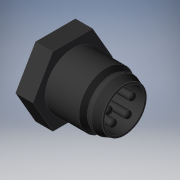
# Autodesk Inventor part: SCHUNK-SNT016581 Stecker EGP
Saved by Autodesk Inventor 2019 (Build 230136000, 136)
## iProperties
Created: 2022-08-29
Part Number: SCHUNK-SNT016581 Stecker EGP
Material: Generic
Catalog Web Link: www.cadenas.de
Description: EGP-Electrical 2-finger parallel gripper
Vendor: SCHUNK
Document SubType Name: Modeling
Designer: psAdmin
Manufacturer: SCHUNK
Mass: 0.444705 g
Surface Area: 5.81753 cm^2
Volume: 0.444705 cm^3
Density: 1 g/cm^3
Appearance: PSOLRGB-175-175-175
Category: PARTsolutions
Company: SCHUNK
Title: SCHUNK-SNT016581 Stecker EGP
Author: Cadenas PARTsolutions
Comments: Electrical 2-finger parallel gripper
PSOL_IDENT_0: {$CADENAS_DATA/23d-libs/schunk/greifsysteme/greifmodule/greifmodule_elektrisch/2_finger_parallelgrei
PSOL_IDENT_1: fer/kleinteilegreifer/egp/egp_stecker.prj},193 {VTYP=3D},{NB=SCHUNK-SNT016581 Stecker EGP},{LINA=SCH
PSOL_IDENT_2: UNK-SNT016581 Stecker EGP},{NN=EGP},{DATE=27.06.2022 11:10:53},{GEOMDATE=04.12.2019 08:06:16},{VERSI
PSOL_IDENT_3: ON=},{LINEID=10},{WBVAR=},{WBNUMERIC=}  {NB=SCHUNK-SNT016581 Stecker EGP},{LINA=SCHUNK-SNT016581 Ste
PSOL_IDENT_4: cker EGP},{KT=DUMMY},{IDNR=SNT016581},{TYP=EGP}
NB: SCHUNK-SNT016581 Stecker EGP
NN: EGP
NT: Electrical 2-finger parallel gripper
NBSYN: SCHUNK-$IDNR. Stecker $TYP.
LINA: SCHUNK-SNT016581 Stecker EGP
CATALOG: SCHUNK
IDNR: SNT016581
TYP: EGP
SUPPLIER: SCHUNK
ARTICLENO: SCHUNK-SNT016581 Stecker EGP
BOMINFO: SCHUNK-SNT016581 Stecker EGP
CREATOR: CADENAS GmbH
Autodesk Inventor part; units mm, degrees
sketch "Sketch_1" plane through (0, 0, 0) normal (0, 0, 1) x (1, 0, 0)
  line L0 (10, 0) -> (0, 0)
  line L1 (0, 0) -> (0, 6)
  line L2 (0, 6) -> (2.5, 6)
  line L3 (2.5, 6) -> (2.5, 4)
  line L4 (2.5, 4) -> (7.4, 4)
  line L5 (7.4, 4) -> (8, 3.4)
  line L6 (8, 3.4) -> (8.5, 3.4)
  line L7 (8.5, 3.4) -> (8.5, 3.6)
  line L8 (8.5, 3.6) -> (8.8, 3.6)
  line L9 (8.8, 3.6) -> (9.9, 3.2)
  line L10 (9.9, 3.2) -> (10, 3.2)
  line L11 (10, 3.2) -> (10, 2.9)
  line L12 (10, 2.9) -> (5, 2.9)
  line L13 (5, 2.9) -> (5, 0)
  line L14 (5, 0) -> (0, 0)
  constraints: 30 end point
revolve "Revolution1" add sketch "Sketch_1" angle 360 about axis through (10, 0, 0) along (1, 0, 0)
sketch "Sketch_2" plane through (0, 0, 0) normal (1, 0, 0) x (0, 1, 0)
  circle A0 centre (0, 0) radius 20
  line L0 (0, 5.7735) -> (-5, 2.8868)
  line L1 (-5, 2.8868) -> (-5, -2.8868)
  line L2 (-5, -2.8868) -> (0, -5.7735)
  line L3 (0, -5.7735) -> (5, -2.8868)
  line L4 (5, -2.8868) -> (5, 2.8868)
  line L5 (5, 2.8868) -> (0, 5.7735)
  constraints: 12 end point, 1 centre point
extrude "Extrusion1" cut sketch "Sketch_2" along normal blind 2.5
sketch "Sketch_3" plane through (0, 0, 1.7) normal (0, 0, 1) x (1, 0, 0)
  line L0 (9.8, 0.5) -> (5, 0.5)
  line L1 (5, 0.5) -> (5, 1)
  line L2 (5, 1) -> (9.3, 1)
  arc A0 (9.8, 0.5) -> (9.3, 1) centre (9.3, 0.5) ccw
  line L3 (9.8, 0.5) -> (5, 0.5)
  constraints: 8 end point, 2 point on circle, 1 centre point
revolve "Revolution2" add sketch "Sketch_3" angle 360 about axis through (9.8, 0.5, 1.7) along (1, 0, 0)
sketch "Pins_SKETCH_1" plane through (0, 0, -1.7) normal (0, 0, 1) x (1, 0, 0)
  line L0 (9.8, 0.5) -> (5, 0.5)
  line L1 (5, 0.5) -> (5, 1)
  line L2 (5, 1) -> (9.3, 1)
  arc A0 (9.8, 0.5) -> (9.3, 1) centre (9.3, 0.5) ccw
  line L3 (9.8, 0.5) -> (5, 0.5)
  constraints: 8 end point, 2 point on circle, 1 centre point
sketch "Pins_SKETCH_2" plane through (0, -1.95, -1.075) normal (0, 0, 1) x (1, 0, 0)
  line L0 (9.8, 0.5) -> (5, 0.5)
  line L1 (5, 0.5) -> (5, 1)
  line L2 (5, 1) -> (9.3, 1)
  arc A0 (9.8, 0.5) -> (9.3, 1) centre (9.3, 0.5) ccw
  line L3 (9.8, 0.5) -> (5, 0.5)
  constraints: 8 end point, 2 point on circle, 1 centre point
sketch "Pins_SKETCH_3" plane through (0, -1.95, 1.075) normal (0, 0, 1) x (1, 0, 0)
  line L0 (9.8, 0.5) -> (5, 0.5)
  line L1 (5, 0.5) -> (5, 1)
  line L2 (5, 1) -> (9.3, 1)
  arc A0 (9.8, 0.5) -> (9.3, 1) centre (9.3, 0.5) ccw
  line L3 (9.8, 0.5) -> (5, 0.5)
  constraints: 8 end point, 2 point on circle, 1 centre point
revolve "Revolution3" add sketch "Pins_SKETCH_1" angle 360 about axis through (9.8, 0.5, -1.7) along (1, 0, 0)
revolve "Revolution4" add sketch "Pins_SKETCH_2" angle 360 about axis through (9.8, -1.45, -1.075) along (1, 0, 0)
revolve "Revolution5" add sketch "Pins_SKETCH_3" angle 360 about axis through (9.8, -1.45, 1.075) along (1, 0, 0)
ref_plane "GEH_XY" through (0, 0, 0) normal (1, 0, 0) x (0, 0, -1)
ref_plane "GEH_YZ" through (0, 0, 0) normal (0, 0, -1) x (0, 1, 0)
ref_plane "GEH_ZX" through (0, 0, 0) normal (0, 1, 0) x (1, 0, 0)
body "Solid1"
